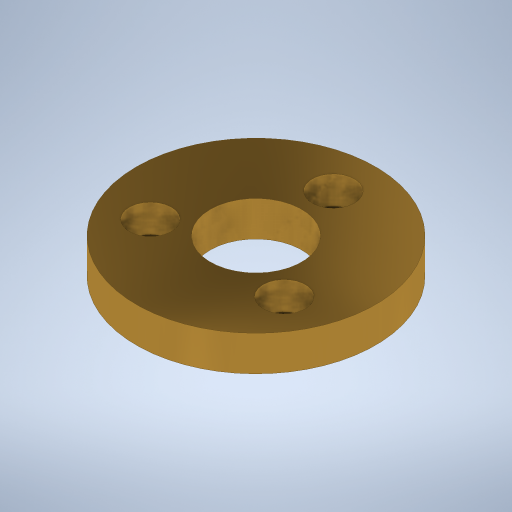
# Autodesk Inventor part: Insert_Top
Saved by Autodesk Inventor 2024 (Build 280153000, 153)
## iProperties
Created: 2023-09-24
Part Number: Insert_Top
Material: Brass
Document SubType Name: Modeling
Designer: schanen
Density: 8.49 g/cm^3
Appearance: Brass - Polished
Author: schanen
Autodesk Inventor part; units mm, degrees
ref_plane "YZ Plane" through (0, 0, 0) normal (1, 0, 0) x (0, 1, 0)
ref_plane "XZ Plane" through (0, 0, 0) normal (0, 1, 0) x (-1, 0, 0)
ref_plane "XY Plane" through (0, 0, 0) normal (0, 0, 1) x (1, 0, 0)
sketch "Sketch1" plane through (0, 0, 0) normal (0, 0, 1) x (1, 0, 0)
  line L0 (-6.5, 0) -> (-17, 0)
  line L1 (-17, 0) -> (-17, 5)
  line L2 (-17, 5) -> (-6.5, 5)
  line L3 (-6.5, 5) -> (-6.5, 0)
  line L4 (0, -1) -> (0, 6) projected
  point P0 (0, 0)
  dimension "d0" = 17
  dimension "d1" = 6.5
  dimension "d2" = 5
  constraints: 8 end point, 2 parallel, 1 horizontal, 1 perpendicular
  measures "d0" distance from line of point (0, 0) L1
  measures "d1" distance from line of point (0, 0) L3
  measures "d2" distance of L0.end L1.end
revolve "Revolution1" add sketch "Sketch1" angle 360 about axis through (0, -10, 0) along (0, 1, 0)
sketch "Sketch3" plane through (0, 5, 0) normal (0, 1, 0) x (1, 0, 0)
  point P0 (0, 0)
  point P1 (0, 11)
  dimension "d16" = 11
  measures "d16" distance of point (0, 0) point (0, 11)
hole "Hole2" at (0, 5, -11) direction (0, -1, 0) diameter 3 end through all counterbore diameter 6 counterbore depth 4
pattern_circular "Circular Pattern1" count 3 over 360 about axis through (0, 2.5, 0) along (0, 1, 0) of "Hole2"
body "Solid1"
